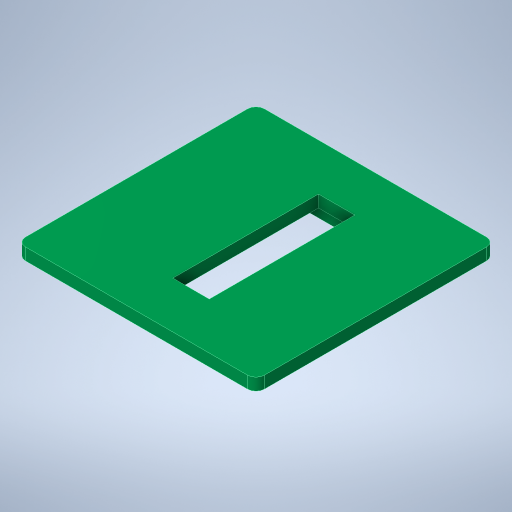
# Autodesk Inventor part: Cover Top (Slotted) Proto
Saved by Autodesk Inventor 2023.1 (Build 271208000, 208)
## iProperties
Created: 2023-02-07
Part Number: Cover Top (Slotted) Proto
Material: Generic
Document SubType Name: Modeling
Designer: xSibe
Density: 1 g/cm^3
Appearance: Plastic Dark Green
Author: xSibe
Autodesk Inventor part; units mm, degrees
ref_plane "YZ Plane" through (0, 0, 0) normal (1, 0, 0) x (0, 1, 0)
ref_plane "XZ Plane" through (0, 0, 0) normal (0, 1, 0) x (-1, 0, 0)
sketch "Sketch1" plane through (0, 0, 0) normal (1, 0, 0) x (0, 1, 0)
  spline S0 degree 2 poles (3.4234, 22.1338) (3.5939, 22.0177) (3.7865, 21.6596) (3.7865, 21.4052) knots 0 0 0 1 2 2 2 projected
  spline S1 degree 2 poles (3.7865, 21.4052) (3.7865, 21.2076) (3.6457, 20.8519) (3.5198, 20.7284) knots 0 0 0 1 2 2 2 projected
  spline S2 degree 2 poles (3.5198, 20.7284) (3.3617, 20.5728) (2.9344, 20.4122) (2.6083, 20.4122) knots 0 0 0 1 2 2 2 projected
  line L0 (2.6083, 20.4122) -> (2.265, 20.4122) projected
  line L1 (2.265, 20.4122) -> (2.265, 19.276) projected
  line L2 (2.265, 19.276) -> (1.8599, 19.276) projected
  line L3 (1.8599, 19.276) -> (1.8599, 22.324) projected
  line L4 (1.8599, 22.324) -> (2.6256, 22.324) projected
  spline S3 degree 2 poles (2.6256, 22.324) (2.8973, 22.324) (3.2777, 22.2351) (3.4234, 22.1338) knots 0 0 0 1 2 2 2 projected
  spline S4 degree 2 poles (0.0667, 22.3882) (0.3779, 22.3882) (0.8769, 22.1709) (1.0498, 21.9757) knots 0 0 0 1 2 2 2 projected
  spline S5 degree 2 poles (1.0498, 21.9757) (1.2227, 21.7732) (1.4153, 21.1804) (1.4153, 20.8) knots 0 0 0 1 2 2 2 projected
  spline S6 degree 2 poles (1.4153, 20.8) (1.4153, 20.4295) (1.2276, 19.8293) (1.0498, 19.6267) knots 0 0 0 1 2 2 2 projected
  spline S7 degree 2 poles (1.0498, 19.6267) (0.862, 19.4143) (0.3656, 19.2118) (0.0667, 19.2118) knots 0 0 0 1 2 2 2 projected
  spline S8 degree 2 poles (0.0667, 19.2118) (-0.2421, 19.2118) (-0.7361, 19.4217) (-0.9164, 19.6267) knots 0 0 0 1 2 2 2 projected
  spline S9 degree 2 poles (-0.9164, 19.6267) (-1.0917, 19.8293) (-1.2795, 20.4246) (-1.2795, 20.8) knots 0 0 0 1 2 2 2 projected
  spline S10 degree 2 poles (-1.2795, 20.8) (-1.2795, 21.1829) (-1.0893, 21.7658) (-0.9139, 21.9757) knots 0 0 0 1 2 2 2 projected
  spline S11 degree 2 poles (-0.9139, 21.9757) (-0.7361, 22.1783) (-0.2396, 22.3882) (0.0667, 22.3882) knots 0 0 0 1 2 2 2 projected
  line L5 (-2.4379, 19.276) -> (-2.843, 19.276) projected
  line L6 (-2.843, 19.276) -> (-2.843, 21.9634) projected
  line L7 (-2.843, 21.9634) -> (-3.8656, 21.9634) projected
  line L8 (-3.8656, 21.9634) -> (-3.8656, 22.324) projected
  line L9 (-3.8656, 22.324) -> (-1.4153, 22.324) projected
  line L10 (-1.4153, 22.324) -> (-1.4153, 21.9634) projected
  line L11 (-1.4153, 21.9634) -> (-2.4379, 21.9634) projected
  line L12 (-2.4379, 21.9634) -> (-2.4379, 19.276) projected
  spline S12 degree 2 poles (22.1338, -3.4234) (22.0177, -3.5939) (21.6596, -3.7865) (21.4052, -3.7865) knots 0 0 0 1 2 2 2 projected
  spline S13 degree 2 poles (21.4052, -3.7865) (21.2076, -3.7865) (20.8519, -3.6457) (20.7284, -3.5198) knots 0 0 0 1 2 2 2 projected
  spline S14 degree 2 poles (20.7284, -3.5198) (20.5728, -3.3617) (20.4122, -2.9344) (20.4122, -2.6083) knots 0 0 0 1 2 2 2 projected
  line L13 (20.4122, -2.6083) -> (20.4122, -2.265) projected
  line L14 (20.4122, -2.265) -> (19.276, -2.265) projected
  line L15 (19.276, -2.265) -> (19.276, -1.8599) projected
  line L16 (19.276, -1.8599) -> (22.324, -1.8599) projected
  line L17 (22.324, -1.8599) -> (22.324, -2.6256) projected
  spline S15 degree 2 poles (22.324, -2.6256) (22.324, -2.8973) (22.2351, -3.2777) (22.1338, -3.4234) knots 0 0 0 1 2 2 2 projected
  spline S16 degree 2 poles (22.3882, -0.0667) (22.3882, -0.3779) (22.1709, -0.8769) (21.9757, -1.0498) knots 0 0 0 1 2 2 2 projected
  spline S17 degree 2 poles (21.9757, -1.0498) (21.7732, -1.2227) (21.1804, -1.4153) (20.8, -1.4153) knots 0 0 0 1 2 2 2 projected
  spline S18 degree 2 poles (20.8, -1.4153) (20.4295, -1.4153) (19.8293, -1.2276) (19.6267, -1.0498) knots 0 0 0 1 2 2 2 projected
  spline S19 degree 2 poles (19.6267, -1.0498) (19.4143, -0.862) (19.2118, -0.3656) (19.2118, -0.0667) knots 0 0 0 1 2 2 2 projected
  spline S20 degree 2 poles (19.2118, -0.0667) (19.2118, 0.2421) (19.4217, 0.7361) (19.6267, 0.9164) knots 0 0 0 1 2 2 2 projected
  spline S21 degree 2 poles (19.6267, 0.9164) (19.8293, 1.0917) (20.4246, 1.2795) (20.8, 1.2795) knots 0 0 0 1 2 2 2 projected
  spline S22 degree 2 poles (20.8, 1.2795) (21.1829, 1.2795) (21.7658, 1.0893) (21.9757, 0.9139) knots 0 0 0 1 2 2 2 projected
  spline S23 degree 2 poles (21.9757, 0.9139) (22.1783, 0.7361) (22.3882, 0.2396) (22.3882, -0.0667) knots 0 0 0 1 2 2 2 projected
  line L18 (19.276, 2.4379) -> (19.276, 2.843) projected
  line L19 (19.276, 2.843) -> (21.9634, 2.843) projected
  line L20 (21.9634, 2.843) -> (21.9634, 3.8656) projected
  line L21 (21.9634, 3.8656) -> (22.324, 3.8656) projected
  line L22 (22.324, 3.8656) -> (22.324, 1.4153) projected
  line L23 (22.324, 1.4153) -> (21.9634, 1.4153) projected
  line L24 (21.9634, 1.4153) -> (21.9634, 2.4379) projected
  line L25 (21.9634, 2.4379) -> (19.276, 2.4379) projected
  spline S24 degree 2 poles (-3.4234, -22.1338) (-3.5939, -22.0177) (-3.7865, -21.6596) (-3.7865, -21.4052) knots 0 0 0 1 2 2 2 projected
  spline S25 degree 2 poles (-3.7865, -21.4052) (-3.7865, -21.2076) (-3.6457, -20.8519) (-3.5198, -20.7284) knots 0 0 0 1 2 2 2 projected
  spline S26 degree 2 poles (-3.5198, -20.7284) (-3.3617, -20.5728) (-2.9344, -20.4122) (-2.6083, -20.4122) knots 0 0 0 1 2 2 2 projected
  line L26 (-2.6083, -20.4122) -> (-2.265, -20.4122) projected
  line L27 (-2.265, -20.4122) -> (-2.265, -19.276) projected
  line L28 (-2.265, -19.276) -> (-1.8599, -19.276) projected
  line L29 (-1.8599, -19.276) -> (-1.8599, -22.324) projected
  line L30 (-1.8599, -22.324) -> (-2.6256, -22.324) projected
  spline S27 degree 2 poles (-2.6256, -22.324) (-2.8973, -22.324) (-3.2777, -22.2351) (-3.4234, -22.1338) knots 0 0 0 1 2 2 2 projected
  spline S28 degree 2 poles (-0.0667, -22.3882) (-0.3779, -22.3882) (-0.8769, -22.1709) (-1.0498, -21.9757) knots 0 0 0 1 2 2 2 projected
  spline S29 degree 2 poles (-1.0498, -21.9757) (-1.2227, -21.7732) (-1.4153, -21.1804) (-1.4153, -20.8) knots 0 0 0 1 2 2 2 projected
  spline S30 degree 2 poles (-1.4153, -20.8) (-1.4153, -20.4295) (-1.2276, -19.8293) (-1.0498, -19.6267) knots 0 0 0 1 2 2 2 projected
  spline S31 degree 2 poles (-1.0498, -19.6267) (-0.862, -19.4143) (-0.3656, -19.2118) (-0.0667, -19.2118) knots 0 0 0 1 2 2 2 projected
  spline S32 degree 2 poles (-0.0667, -19.2118) (0.2421, -19.2118) (0.7361, -19.4217) (0.9164, -19.6267) knots 0 0 0 1 2 2 2 projected
  spline S33 degree 2 poles (0.9164, -19.6267) (1.0917, -19.8293) (1.2795, -20.4246) (1.2795, -20.8) knots 0 0 0 1 2 2 2 projected
  spline S34 degree 2 poles (1.2795, -20.8) (1.2795, -21.1829) (1.0893, -21.7658) (0.9139, -21.9757) knots 0 0 0 1 2 2 2 projected
  spline S35 degree 2 poles (0.9139, -21.9757) (0.7361, -22.1783) (0.2396, -22.3882) (-0.0667, -22.3882) knots 0 0 0 1 2 2 2 projected
  line L31 (2.4379, -19.276) -> (2.843, -19.276) projected
  line L32 (2.843, -19.276) -> (2.843, -21.9634) projected
  line L33 (2.843, -21.9634) -> (3.8656, -21.9634) projected
  line L34 (3.8656, -21.9634) -> (3.8656, -22.324) projected
  line L35 (3.8656, -22.324) -> (1.4153, -22.324) projected
  line L36 (1.4153, -22.324) -> (1.4153, -21.9634) projected
  line L37 (1.4153, -21.9634) -> (2.4379, -21.9634) projected
  line L38 (2.4379, -21.9634) -> (2.4379, -19.276) projected
  spline S36 degree 2 poles (-22.1338, 3.4234) (-22.0177, 3.5939) (-21.6596, 3.7865) (-21.4052, 3.7865) knots 0 0 0 1 2 2 2 projected
  spline S37 degree 2 poles (-21.4052, 3.7865) (-21.2076, 3.7865) (-20.8519, 3.6457) (-20.7284, 3.5198) knots 0 0 0 1 2 2 2 projected
  spline S38 degree 2 poles (-20.7284, 3.5198) (-20.5728, 3.3617) (-20.4122, 2.9344) (-20.4122, 2.6083) knots 0 0 0 1 2 2 2 projected
  line L39 (-20.4122, 2.6083) -> (-20.4122, 2.265) projected
  line L40 (-20.4122, 2.265) -> (-19.276, 2.265) projected
  line L41 (-19.276, 2.265) -> (-19.276, 1.8599) projected
  line L42 (-19.276, 1.8599) -> (-22.324, 1.8599) projected
  line L43 (-22.324, 1.8599) -> (-22.324, 2.6256) projected
  spline S39 degree 2 poles (-22.324, 2.6256) (-22.324, 2.8973) (-22.2351, 3.2777) (-22.1338, 3.4234) knots 0 0 0 1 2 2 2 projected
  spline S40 degree 2 poles (-22.3882, 0.0667) (-22.3882, 0.3779) (-22.1709, 0.8769) (-21.9757, 1.0498) knots 0 0 0 1 2 2 2 projected
  spline S41 degree 2 poles (-21.9757, 1.0498) (-21.7732, 1.2227) (-21.1804, 1.4153) (-20.8, 1.4153) knots 0 0 0 1 2 2 2 projected
  spline S42 degree 2 poles (-20.8, 1.4153) (-20.4295, 1.4153) (-19.8293, 1.2276) (-19.6267, 1.0498) knots 0 0 0 1 2 2 2 projected
  spline S43 degree 2 poles (-19.6267, 1.0498) (-19.4143, 0.862) (-19.2118, 0.3656) (-19.2118, 0.0667) knots 0 0 0 1 2 2 2 projected
  spline S44 degree 2 poles (-19.2118, 0.0667) (-19.2118, -0.2421) (-19.4217, -0.7361) (-19.6267, -0.9164) knots 0 0 0 1 2 2 2 projected
  spline S45 degree 2 poles (-19.6267, -0.9164) (-19.8293, -1.0917) (-20.4246, -1.2795) (-20.8, -1.2795) knots 0 0 0 1 2 2 2 projected
  spline S46 degree 2 poles (-20.8, -1.2795) (-21.1829, -1.2795) (-21.7658, -1.0893) (-21.9757, -0.9139) knots 0 0 0 1 2 2 2 projected
  spline S47 degree 2 poles (-21.9757, -0.9139) (-22.1783, -0.7361) (-22.3882, -0.2396) (-22.3882, 0.0667) knots 0 0 0 1 2 2 2 projected
  line L44 (-19.276, -2.4379) -> (-19.276, -2.843) projected
  line L45 (-19.276, -2.843) -> (-21.9634, -2.843) projected
  line L46 (-21.9634, -2.843) -> (-21.9634, -3.8656) projected
  line L47 (-21.9634, -3.8656) -> (-22.324, -3.8656) projected
  line L48 (-22.324, -3.8656) -> (-22.324, -1.4153) projected
  line L49 (-22.324, -1.4153) -> (-21.9634, -1.4153) projected
  line L50 (-21.9634, -1.4153) -> (-21.9634, -2.4379) projected
  line L51 (-21.9634, -2.4379) -> (-19.276, -2.4379) projected
  circle A0 centre (-21.9, 21.9) radius 1.875 projected
  circle A1 centre (21.9, -21.9) radius 1.875 projected
  circle A2 centre (-21.9, -21.9) radius 1.875 projected
  circle A3 centre (21.9, 21.9) radius 1.875 projected
  circle A4 centre (20.8, -14.4) radius 2.0788 projected
  circle A5 centre (-20.8, 14.4) radius 2.0788 projected
  circle A6 centre (-20.8, -14.4) radius 2.0788 projected
  circle A7 centre (-14.4, -20.8) radius 2.0788 projected
  line L52 (17.05, 17.05) -> (-17.05, 17.05) projected
  line L53 (17.05, -17.05) -> (17.05, 17.05) projected
  line L54 (-17.05, -17.05) -> (17.05, -17.05) projected
  line L55 (-17.05, 17.05) -> (-17.05, -17.05) projected
  circle A8 centre (14.4, -20.8) radius 2.0788 projected
  circle A9 centre (20.8, 14.4) radius 2.0788 projected
  circle A10 centre (-14.4, 20.8) radius 2.0788 projected
  circle A11 centre (14.4, 20.8) radius 2.0788 projected
  line L56 (24.875, 22.9) -> (24.875, -22.9) projected
  arc A12 (24.875, 22.9) -> (22.9, 24.875) centre (22.9, 22.9) ccw projected
  line L57 (-22.9, 24.875) -> (22.9, 24.875) projected
  arc A13 (-22.9, 24.875) -> (-24.875, 22.9) centre (-22.9, 22.9) ccw projected
  line L58 (-24.875, -22.9) -> (-24.875, 22.9) projected
  arc A14 (-24.875, -22.9) -> (-22.9, -24.875) centre (-22.9, -22.9) ccw projected
  line L59 (22.9, -24.875) -> (-22.9, -24.875) projected
  arc A15 (22.9, -24.875) -> (24.875, -22.9) centre (22.9, -22.9) ccw projected
  arc A16 (-24.625, -22.9) -> (-22.9, -24.625) centre (-22.9, -22.9) ccw
  line L60 (-24.625, -22.9) -> (-24.625, 22.9)
  arc A17 (-22.9, 24.625) -> (-24.625, 22.9) centre (-22.9, 22.9) ccw
  line L61 (-22.9, 24.625) -> (22.9, 24.625)
  arc A18 (24.625, 22.9) -> (22.9, 24.625) centre (22.9, 22.9) ccw
  line L62 (24.625, 22.9) -> (24.625, -22.9)
  arc A19 (22.9, -24.625) -> (24.625, -22.9) centre (22.9, -22.9) ccw
  line L63 (22.9, -24.625) -> (-22.9, -24.625)
  point P0 (0, 0)
  dimension "d0" = 0.25
  constraints: 8 end point, 8 point on circle, 4 centre point, 7 other
  measures "d0" distance between parallel lines of L59 L63
ref_plane "Work Plane1" through (49.8, -24.875, -24.875) normal (1, 0, 0) x (0, 1, 0)
extrude "Extrusion1" add sketch "Sketch1" along normal blind 2.5 from surface at 49.8 contours S0 S1 S2 L0 L1 L2 L3 L4 S3 | S4 S5 S6 S7 S8 S9 S10 S11 | L5 L6 L7 L8 L9 L10 L11 L12 | S12 S13 S14 L13 L14 L15 L16 L17 S15 | S16 S17 S18 S19 S20 S21 S22 S23 | L18 L19 L20 L21 L22 L23 L24 L25 | S24 S25 S26 L26 L27 L28 L29 L30 S27 | S28 S29 S30 S31 S32 S33 S34 S35 | L31 L32 L33 L34 L35 L36 L37 L38 | S36 S37 S38 L39 L40 L41 L42 L43 S39 | S40 S41 S42 S43 S44 S45 S46 S47 | L44 L45 L46 L47 L48 L49 L50 L51 | A0 | A1 | A2 | A3 | A4 | A5 | A6 | A7 | L53 L54 L55 L52 | A8 | A9 | A10 | A11 | L60 A17 L61 A18 L62 A19 L63 A16
sketch "Sketch2" plane through (52.3, -22.9, -24.625) normal (1, 0, 0) x (0, 0, -1)
  spline S0 degree 2 poles (-46.7588, 26.3234) (-46.6427, 26.4939) (-46.2846, 26.6865) (-46.0302, 26.6865) knots 0 0 0 1 2 2 2 projected
  spline S1 degree 2 poles (-46.0302, 26.6865) (-45.8326, 26.6865) (-45.4769, 26.5457) (-45.3534, 26.4198) knots 0 0 0 1 2 2 2 projected
  spline S2 degree 2 poles (-45.3534, 26.4198) (-45.1978, 26.2617) (-45.0372, 25.8344) (-45.0372, 25.5083) knots 0 0 0 1 2 2 2 projected
  line L0 (-45.0372, 25.5083) -> (-45.0372, 25.165) projected
  line L1 (-45.0372, 25.165) -> (-43.901, 25.165) projected
  line L2 (-43.901, 25.165) -> (-43.901, 24.7599) projected
  line L3 (-43.901, 24.7599) -> (-46.949, 24.7599) projected
  line L4 (-46.949, 24.7599) -> (-46.949, 25.5256) projected
  spline S3 degree 2 poles (-46.949, 25.5256) (-46.949, 25.7973) (-46.8601, 26.1777) (-46.7588, 26.3234) knots 0 0 0 1 2 2 2 projected
  spline S4 degree 2 poles (-47.0132, 22.9667) (-47.0132, 23.2779) (-46.7959, 23.7769) (-46.6007, 23.9498) knots 0 0 0 1 2 2 2 projected
  spline S5 degree 2 poles (-46.6007, 23.9498) (-46.3982, 24.1227) (-45.8054, 24.3153) (-45.425, 24.3153) knots 0 0 0 1 2 2 2 projected
  spline S6 degree 2 poles (-45.425, 24.3153) (-45.0545, 24.3153) (-44.4543, 24.1276) (-44.2517, 23.9498) knots 0 0 0 1 2 2 2 projected
  spline S7 degree 2 poles (-44.2517, 23.9498) (-44.0393, 23.762) (-43.8368, 23.2656) (-43.8368, 22.9667) knots 0 0 0 1 2 2 2 projected
  spline S8 degree 2 poles (-43.8368, 22.9667) (-43.8368, 22.6579) (-44.0467, 22.1639) (-44.2517, 21.9836) knots 0 0 0 1 2 2 2 projected
  spline S9 degree 2 poles (-44.2517, 21.9836) (-44.4543, 21.8083) (-45.0496, 21.6205) (-45.425, 21.6205) knots 0 0 0 1 2 2 2 projected
  spline S10 degree 2 poles (-45.425, 21.6205) (-45.8079, 21.6205) (-46.3908, 21.8107) (-46.6007, 21.9861) knots 0 0 0 1 2 2 2 projected
  spline S11 degree 2 poles (-46.6007, 21.9861) (-46.8033, 22.1639) (-47.0132, 22.6604) (-47.0132, 22.9667) knots 0 0 0 1 2 2 2 projected
  line L5 (-43.901, 20.4621) -> (-43.901, 20.057) projected
  line L6 (-43.901, 20.057) -> (-46.5884, 20.057) projected
  line L7 (-46.5884, 20.057) -> (-46.5884, 19.0344) projected
  line L8 (-46.5884, 19.0344) -> (-46.949, 19.0344) projected
  line L9 (-46.949, 19.0344) -> (-46.949, 21.4847) projected
  line L10 (-46.949, 21.4847) -> (-46.5884, 21.4847) projected
  line L11 (-46.5884, 21.4847) -> (-46.5884, 20.4621) projected
  line L12 (-46.5884, 20.4621) -> (-43.901, 20.4621) projected
  spline S12 degree 2 poles (-21.2016, 45.0338) (-21.0311, 44.9177) (-20.8385, 44.5596) (-20.8385, 44.3052) knots 0 0 0 1 2 2 2 projected
  spline S13 degree 2 poles (-20.8385, 44.3052) (-20.8385, 44.1076) (-20.9793, 43.7519) (-21.1052, 43.6284) knots 0 0 0 1 2 2 2 projected
  spline S14 degree 2 poles (-21.1052, 43.6284) (-21.2633, 43.4728) (-21.6906, 43.3122) (-22.0167, 43.3122) knots 0 0 0 1 2 2 2 projected
  line L13 (-22.0167, 43.3122) -> (-22.36, 43.3122) projected
  line L14 (-22.36, 43.3122) -> (-22.36, 42.176) projected
  line L15 (-22.36, 42.176) -> (-22.7651, 42.176) projected
  line L16 (-22.7651, 42.176) -> (-22.7651, 45.224) projected
  line L17 (-22.7651, 45.224) -> (-21.9994, 45.224) projected
  spline S15 degree 2 poles (-21.9994, 45.224) (-21.7277, 45.224) (-21.3473, 45.1351) (-21.2016, 45.0338) knots 0 0 0 1 2 2 2 projected
  spline S16 degree 2 poles (-24.5583, 45.2882) (-24.2471, 45.2882) (-23.7481, 45.0709) (-23.5752, 44.8757) knots 0 0 0 1 2 2 2 projected
  spline S17 degree 2 poles (-23.5752, 44.8757) (-23.4023, 44.6732) (-23.2097, 44.0804) (-23.2097, 43.7) knots 0 0 0 1 2 2 2 projected
  spline S18 degree 2 poles (-23.2097, 43.7) (-23.2097, 43.3295) (-23.3974, 42.7293) (-23.5752, 42.5267) knots 0 0 0 1 2 2 2 projected
  spline S19 degree 2 poles (-23.5752, 42.5267) (-23.763, 42.3143) (-24.2594, 42.1118) (-24.5583, 42.1118) knots 0 0 0 1 2 2 2 projected
  spline S20 degree 2 poles (-24.5583, 42.1118) (-24.8671, 42.1118) (-25.3611, 42.3217) (-25.5414, 42.5267) knots 0 0 0 1 2 2 2 projected
  spline S21 degree 2 poles (-25.5414, 42.5267) (-25.7167, 42.7293) (-25.9045, 43.3246) (-25.9045, 43.7) knots 0 0 0 1 2 2 2 projected
  spline S22 degree 2 poles (-25.9045, 43.7) (-25.9045, 44.0829) (-25.7143, 44.6658) (-25.5389, 44.8757) knots 0 0 0 1 2 2 2 projected
  spline S23 degree 2 poles (-25.5389, 44.8757) (-25.3611, 45.0783) (-24.8646, 45.2882) (-24.5583, 45.2882) knots 0 0 0 1 2 2 2 projected
  line L18 (-27.0629, 42.176) -> (-27.468, 42.176) projected
  line L19 (-27.468, 42.176) -> (-27.468, 44.8634) projected
  line L20 (-27.468, 44.8634) -> (-28.4906, 44.8634) projected
  line L21 (-28.4906, 44.8634) -> (-28.4906, 45.224) projected
  line L22 (-28.4906, 45.224) -> (-26.0403, 45.224) projected
  line L23 (-26.0403, 45.224) -> (-26.0403, 44.8634) projected
  line L24 (-26.0403, 44.8634) -> (-27.0629, 44.8634) projected
  line L25 (-27.0629, 44.8634) -> (-27.0629, 42.176) projected
  spline S24 degree 2 poles (-2.4912, 19.4766) (-2.6073, 19.3061) (-2.9654, 19.1135) (-3.2198, 19.1135) knots 0 0 0 1 2 2 2 projected
  spline S25 degree 2 poles (-3.2198, 19.1135) (-3.4174, 19.1135) (-3.7731, 19.2543) (-3.8966, 19.3802) knots 0 0 0 1 2 2 2 projected
  spline S26 degree 2 poles (-3.8966, 19.3802) (-4.0522, 19.5383) (-4.2128, 19.9656) (-4.2128, 20.2917) knots 0 0 0 1 2 2 2 projected
  line L26 (-4.2128, 20.2917) -> (-4.2128, 20.635) projected
  line L27 (-4.2128, 20.635) -> (-5.349, 20.635) projected
  line L28 (-5.349, 20.635) -> (-5.349, 21.0401) projected
  line L29 (-5.349, 21.0401) -> (-2.301, 21.0401) projected
  line L30 (-2.301, 21.0401) -> (-2.301, 20.2744) projected
  spline S27 degree 2 poles (-2.301, 20.2744) (-2.301, 20.0027) (-2.3899, 19.6223) (-2.4912, 19.4766) knots 0 0 0 1 2 2 2 projected
  spline S28 degree 2 poles (-2.2368, 22.8333) (-2.2368, 22.5221) (-2.4541, 22.0231) (-2.6493, 21.8502) knots 0 0 0 1 2 2 2 projected
  spline S29 degree 2 poles (-2.6493, 21.8502) (-2.8518, 21.6773) (-3.4446, 21.4847) (-3.825, 21.4847) knots 0 0 0 1 2 2 2 projected
  spline S30 degree 2 poles (-3.825, 21.4847) (-4.1955, 21.4847) (-4.7957, 21.6724) (-4.9983, 21.8502) knots 0 0 0 1 2 2 2 projected
  spline S31 degree 2 poles (-4.9983, 21.8502) (-5.2107, 22.038) (-5.4132, 22.5344) (-5.4132, 22.8333) knots 0 0 0 1 2 2 2 projected
  spline S32 degree 2 poles (-5.4132, 22.8333) (-5.4132, 23.1421) (-5.2033, 23.6361) (-4.9983, 23.8164) knots 0 0 0 1 2 2 2 projected
  spline S33 degree 2 poles (-4.9983, 23.8164) (-4.7957, 23.9917) (-4.2004, 24.1795) (-3.825, 24.1795) knots 0 0 0 1 2 2 2 projected
  spline S34 degree 2 poles (-3.825, 24.1795) (-3.4421, 24.1795) (-2.8592, 23.9893) (-2.6493, 23.8139) knots 0 0 0 1 2 2 2 projected
  spline S35 degree 2 poles (-2.6493, 23.8139) (-2.4467, 23.6361) (-2.2368, 23.1396) (-2.2368, 22.8333) knots 0 0 0 1 2 2 2 projected
  line L31 (-5.349, 25.3379) -> (-5.349, 25.743) projected
  line L32 (-5.349, 25.743) -> (-2.6616, 25.743) projected
  line L33 (-2.6616, 25.743) -> (-2.6616, 26.7656) projected
  line L34 (-2.6616, 26.7656) -> (-2.301, 26.7656) projected
  line L35 (-2.301, 26.7656) -> (-2.301, 24.3153) projected
  line L36 (-2.301, 24.3153) -> (-2.6616, 24.3153) projected
  line L37 (-2.6616, 24.3153) -> (-2.6616, 25.3379) projected
  line L38 (-2.6616, 25.3379) -> (-5.349, 25.3379) projected
  spline S36 degree 2 poles (-28.0484, 0.7662) (-28.2189, 0.8823) (-28.4115, 1.2404) (-28.4115, 1.4948) knots 0 0 0 1 2 2 2 projected
  spline S37 degree 2 poles (-28.4115, 1.4948) (-28.4115, 1.6924) (-28.2707, 2.0481) (-28.1448, 2.1716) knots 0 0 0 1 2 2 2 projected
  spline S38 degree 2 poles (-28.1448, 2.1716) (-27.9867, 2.3272) (-27.5594, 2.4878) (-27.2333, 2.4878) knots 0 0 0 1 2 2 2 projected
  line L39 (-27.2333, 2.4878) -> (-26.89, 2.4878) projected
  line L40 (-26.89, 2.4878) -> (-26.89, 3.624) projected
  line L41 (-26.89, 3.624) -> (-26.4849, 3.624) projected
  line L42 (-26.4849, 3.624) -> (-26.4849, 0.576) projected
  line L43 (-26.4849, 0.576) -> (-27.2506, 0.576) projected
  spline S39 degree 2 poles (-27.2506, 0.576) (-27.5223, 0.576) (-27.9027, 0.6649) (-28.0484, 0.7662) knots 0 0 0 1 2 2 2 projected
  spline S40 degree 2 poles (-24.6917, 0.5118) (-25.0029, 0.5118) (-25.5019, 0.7291) (-25.6748, 0.9243) knots 0 0 0 1 2 2 2 projected
  spline S41 degree 2 poles (-25.6748, 0.9243) (-25.8477, 1.1268) (-26.0403, 1.7196) (-26.0403, 2.1) knots 0 0 0 1 2 2 2 projected
  spline S42 degree 2 poles (-26.0403, 2.1) (-26.0403, 2.4705) (-25.8526, 3.0707) (-25.6748, 3.2733) knots 0 0 0 1 2 2 2 projected
  spline S43 degree 2 poles (-25.6748, 3.2733) (-25.487, 3.4857) (-24.9906, 3.6882) (-24.6917, 3.6882) knots 0 0 0 1 2 2 2 projected
  spline S44 degree 2 poles (-24.6917, 3.6882) (-24.3829, 3.6882) (-23.8889, 3.4783) (-23.7086, 3.2733) knots 0 0 0 1 2 2 2 projected
  spline S45 degree 2 poles (-23.7086, 3.2733) (-23.5333, 3.0707) (-23.3455, 2.4754) (-23.3455, 2.1) knots 0 0 0 1 2 2 2 projected
  spline S46 degree 2 poles (-23.3455, 2.1) (-23.3455, 1.7171) (-23.5357, 1.1342) (-23.7111, 0.9243) knots 0 0 0 1 2 2 2 projected
  spline S47 degree 2 poles (-23.7111, 0.9243) (-23.8889, 0.7217) (-24.3854, 0.5118) (-24.6917, 0.5118) knots 0 0 0 1 2 2 2 projected
  line L44 (-22.1871, 3.624) -> (-21.782, 3.624) projected
  line L45 (-21.782, 3.624) -> (-21.782, 0.9366) projected
  line L46 (-21.782, 0.9366) -> (-20.7594, 0.9366) projected
  line L47 (-20.7594, 0.9366) -> (-20.7594, 0.576) projected
  line L48 (-20.7594, 0.576) -> (-23.2097, 0.576) projected
  line L49 (-23.2097, 0.576) -> (-23.2097, 0.9366) projected
  line L50 (-23.2097, 0.9366) -> (-22.1871, 0.9366) projected
  line L51 (-22.1871, 0.9366) -> (-22.1871, 3.624) projected
  circle A0 centre (-46.525, 1) radius 1.875 projected
  circle A1 centre (-2.725, 44.8) radius 1.875 projected
  circle A2 centre (-2.725, 1) radius 1.875 projected
  circle A3 centre (-46.525, 44.8) radius 1.875 projected
  circle A4 centre (-10.225, 43.7) radius 2.0788 projected
  circle A5 centre (-39.025, 2.1) radius 2.0788 projected
  circle A6 centre (-10.225, 2.1) radius 2.0788 projected
  circle A7 centre (-3.825, 8.5) radius 2.0788 projected
  line L52 (-41.675, 39.95) -> (-41.675, 5.85) projected
  line L53 (-7.575, 39.95) -> (-41.675, 39.95) projected
  line L54 (-7.575, 5.85) -> (-7.575, 39.95) projected
  line L55 (-41.675, 5.85) -> (-7.575, 5.85) projected
  circle A8 centre (-3.825, 37.3) radius 2.0788 projected
  circle A9 centre (-39.025, 43.7) radius 2.0788 projected
  circle A10 centre (-45.425, 8.5) radius 2.0788 projected
  circle A11 centre (-45.425, 37.3) radius 2.0788 projected
  line L56 (-47.525, 47.775) -> (-1.725, 47.775) projected
  arc A12 (-47.525, 47.775) -> (-49.5, 45.8) centre (-47.525, 45.8) ccw projected
  line L57 (-49.5, 0) -> (-49.5, 45.8) projected
  arc A13 (-49.5, 0) -> (-47.525, -1.975) centre (-47.525, 0) ccw projected
  line L58 (-1.725, -1.975) -> (-47.525, -1.975) projected
  arc A14 (-1.725, -1.975) -> (0.25, 0) centre (-1.725, 0) ccw projected
  line L59 (0.25, 45.8) -> (0.25, 0) projected
  arc A15 (0.25, 45.8) -> (-1.725, 47.775) centre (-1.725, 45.8) ccw projected
  circle A16 centre (-2.725, 44.8) radius 1.8
  circle A17 centre (-2.725, 1) radius 1.8
  circle A18 centre (-46.525, 1) radius 1.8
  circle A19 centre (-46.525, 44.8) radius 1.8
  line L60 (-7.65, 39.875) -> (-41.6, 39.875)
  line L61 (-41.6, 39.875) -> (-41.6, 5.925)
  line L62 (-41.6, 5.925) -> (-7.65, 5.925)
  line L63 (-7.65, 5.925) -> (-7.65, 39.875)
  line L64 (-8.9, 38.625) -> (-40.35, 38.625)
  line L65 (-40.35, 38.625) -> (-40.35, 7.175)
  line L66 (-40.35, 7.175) -> (-8.9, 7.175)
  line L67 (-8.9, 7.175) -> (-8.9, 38.625)
  point P0 (-24.625, 22.9)
  dimension "d3" = 0.075
  dimension "d4" = 0.075
  dimension "d5" = 0.075
  dimension "d6" = 0.075
  dimension "d20" = 0.075
  dimension "d21" = 1.25
  constraints: 16 end point, 4 centre point, 6 other
  measures "d3" radial gap between concentric circles of A1 A16
  measures "d4" radial gap between concentric circles of A2 A17
  measures "d5" radial gap between concentric circles of A0 A18
  measures "d6" radial gap between concentric circles of A3 A19
  measures "d20" distance between parallel lines of L54 L63
  measures "d21" distance between parallel lines of L63 L67
extrude "Extrusion2" add sketch "Sketch2" against normal blind 2.5 from surface at -2.5 contours L63 L62 L61 L60
sketch "Sketch3" plane through (52.3, -22.9, -24.625) normal (1, 0, 0) x (0, 0, -1)
  arc A0 (-49.25, 0) -> (-47.525, -1.725) centre (-47.525, 0) ccw projected
  line L0 (-1.725, -1.725) -> (-47.525, -1.725) projected
  arc A1 (-1.725, -1.725) -> (0, 0) centre (-1.725, 0) ccw projected
  line L1 (0, 45.8) -> (0, 0) projected
  arc A2 (0, 45.8) -> (-1.725, 47.525) centre (-1.725, 45.8) ccw projected
  line L2 (-47.525, 47.525) -> (-1.725, 47.525) projected
  arc A3 (-47.525, 47.525) -> (-49.25, 45.8) centre (-47.525, 45.8) ccw projected
  line L3 (-49.25, 0) -> (-49.25, 45.8) projected
  line L4 (-24.625, -1.725) -> (-24.625, 21.275)
  line L5 (-39.625, 25.025) -> (-9.625, 25.025)
  line L6 (-9.625, 25.025) -> (-9.625, 17.525)
  line L7 (-9.625, 17.525) -> (-39.625, 17.525)
  line L8 (-39.625, 17.525) -> (-39.625, 25.025)
  line L9 (-39.625, 25.025) -> (-9.625, 17.525) construction
  line L10 (-9.625, 25.025) -> (-39.625, 17.525) construction
  point P0 (-24.625, 22.9)
  dimension "d12" = 23
  dimension "d13" = 30
  dimension "d14" = 7.5
  constraints: 14 end point, 3 midpoint, 2 parallel, 1 horizontal, 1 perpendicular, 1 vertical
  measures "d12" distance of L4.start L4.end
  measures "d13" distance of L6.end L7.end
  measures "d14" distance of L5.end L6.end
extrude "Extrusion3" cut sketch "Sketch3" against normal up to surface (2.5 mm away) contours L7 L8 L5 L6
body "Solid1"
